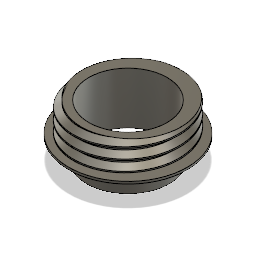
adapter (Autodesk Fusion 360 design; units mm, degrees)
Autodesk Fusion 360 part; units mm, degrees
sketch "Sketch1" plane through (0, 0, 0) normal (0, 1, 0) x (1, 0, 0)
  circle A0 centre (0, 0) radius 17.55
  circle A1 centre (0, 0) radius 16.55
  dimension "d1" = 35.1
  dimension "d2" = -1
  constraint coincident A0.centre A1.centre
  measures "d1" diameter of A0
extrude "Extrude1" add sketch "Sketch1" along normal blind 10
sketch "Sketch2" plane through (0, 10, 0) normal (0, 1, 0) x (-1, 0, 0)
  circle A0 centre (0, 0) radius 16.55
  circle A1 centre (0, 0) radius 17.55
  circle A2 centre (0, 0) radius 25.2
  circle A3 centre (0, 0) radius 26.2
  dimension "d5" = 50.4
  dimension "d6" = 1
  constraint concentric A0 A2
  measures "d5" diameter of A2
extrude "Extrude4" add sketch "Sketch2" along normal blind 1 from surface at -1 contours A2
sketch "Sketch7" plane through (0, 10, 0) normal (0, 1, 0) x (-1, 0, 0)
  circle A0 centre (0, 0) radius 25.2
  circle A1 centre (0, 0) radius 16.55
  circle A2 centre (0, 0) radius 21.9
  dimension "d17" = 43.8
  constraint concentric A0 A2
  measures "d17" diameter of A2
extrude "Extrude5" add sketch "Sketch7" along normal blind 12 contours A2
thread "Thread3" "ISO Metric profile 45.0 M45x4.5 6g" major diameter 44.687 minor diameter 39.5358 pitch 4.5 angle 60 modelled right hand crest width 0.5625 on face at (-21.8728, 18, -1.0916) crest through (-22.3435, 9.7188, 0)
equation "d1 = 36 mm - 0.4 mm - 0.5 mm"
equation "d17 = 44 mm - 0.2 mm"
